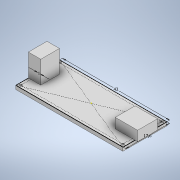
# Autodesk Inventor part: nano_footprint
Saved by Autodesk Inventor 2021 (Build 250183000, 183)
## iProperties
Created: 2021-12-12
Part Number: nano_footprint
Material: Generic
Document SubType Name: Modeling
Designer: Juan M. Casillas
Density: 1 g/cm^3
Appearance: Default
Author: Juan M. Casillas
Autodesk Inventor part; units mm, degrees
ref_plane "YZ Plane" through (0, 0, 0) normal (1, 0, 0) x (0, 1, 0)
ref_plane "XZ Plane" through (0, 0, 0) normal (0, 1, 0) x (-1, 0, 0)
ref_plane "XY Plane" through (0, 0, 0) normal (0, 0, 1) x (1, 0, 0)
sketch "Sketch1" plane through (0, 0, 0) normal (0, 1, 0) x (-1, 0, 0)
  line L0 (21.5, 8.8) -> (-21.5, 8.8)
  line L1 (-21.5, 8.8) -> (-21.5, -8.8)
  line L2 (-21.5, -8.8) -> (21.5, -8.8)
  line L3 (21.5, -8.8) -> (21.5, 8.8)
  line L4 (21.5, 8.8) -> (-21.5, -8.8) construction
  line L5 (-21.5, 8.8) -> (21.5, -8.8) construction
  line L6 (20.5, 7.8) -> (-20.5, 7.8) construction
  line L7 (-20.5, 7.8) -> (-20.5, -7.8) construction
  line L8 (-20.5, -7.8) -> (20.5, -7.8) construction
  line L9 (20.5, -7.8) -> (20.5, 7.8) construction
  point P0 (0, 0)
  dimension "d0" = 43
  dimension "d1" = 17.6
  dimension "d2" = 1
  constraints: 20 end point, 4 coincident, 4 parallel, 2 midpoint, 2 perpendicular, 1 horizontal, 3 other
  measures "d0" distance of L2.end L1.end
  measures "d1" distance of L1.end L0.end
  measures "d2" distance between parallel lines of L3 L9
extrude "Extrusion1" add sketch "Sketch1" against normal blind 1.5
hole "Hole1" at (-20.5, 0, 7.8) at (-20.5, 0, -7.8) at (20.5, 0, 7.8) at (20.5, 0, -7.8) direction (0, -1, 0) diameter 1 end through all
sketch "Sketch2" plane through (0, 0, 0) normal (0, 1, 0) x (1, 0, 0)
  line L0 (-21.5, 3.75) -> (-16.5, 3.75)
  line L1 (-16.5, 3.75) -> (-16.5, -3.75)
  line L2 (-16.5, -3.75) -> (-21.5, -3.75)
  line L3 (-21.5, -3.75) -> (-21.5, 3.75)
  line L4 (-21.5, 3.75) -> (-16.5, -3.75) construction
  line L5 (-16.5, 3.75) -> (-21.5, -3.75) construction
  line L6 (-21.5, 8.8) -> (-21.5, -8.8) projected
  point P0 (0, 0)
  point P1 (-19, 0)
  point P2 (-21.5, 0)
  dimension "d12" = 5
  dimension "d13" = 7.5
  constraints: 12 end point, 4 midpoint, 2 parallel, 1 horizontal, 1 perpendicular
  measures "d12" distance of L1.end L2.end
  measures "d13" distance of L0.end L1.end
extrude "Extrusion2" add sketch "Sketch2" along normal blind 9
sketch "Sketch3" plane through (0, 0, 0) normal (0, 1, 0) x (1, 0, 0)
  point P0 (0, 0)
sketch "Sketch4" plane through (0, 0, 0) normal (0, 1, 0) x (1, 0, 0)
  line L0 (13.6557, 4) -> (22.6557, 4)
  line L1 (22.6557, 4) -> (22.6557, -4)
  line L2 (22.6557, -4) -> (13.6557, -4)
  line L3 (13.6557, -4) -> (13.6557, 4)
  line L4 (13.6557, 4) -> (22.6557, -4) construction
  line L5 (22.6557, 4) -> (13.6557, -4) construction
  point P0 (0, 0)
  point P1 (18.1557, 0)
  dimension "d16" = 9
  dimension "d17" = 8
  constraints: 12 end point, 2 midpoint, 2 parallel, 1 horizontal, 1 perpendicular
  measures "d16" distance of L1.end L2.end
  measures "d17" distance of L0.end L1.end
extrude "Extrusion3" add sketch "Sketch4" along normal blind 4
body "Solid1"
